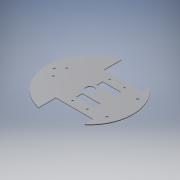
# Autodesk Inventor part: Base Inferior
Saved by Autodesk Inventor 2017 (Build 210142000, 142)
## iProperties
Created: 2017-08-05
Part Number: Base Inferior
Material: Glass
Document SubType Name: Modeling
Designer: Andre Rodas
Density: 2.18 g/cm^3
Appearance: Clear
Author: Andre Rodas
Autodesk Inventor part; units mm, degrees
ref_plane "YZ Plane" through (0, 0, 0) normal (1, 0, 0) x (0, 1, 0)
ref_plane "XZ Plane" through (0, 0, 0) normal (0, 1, 0) x (-1, 0, 0)
ref_plane "XY Plane" through (0, 0, 0) normal (0, 0, 1) x (1, 0, 0)
sketch "Sketch1" plane through (0, 0, 0) normal (0, 0, 1) x (1, 0, 0)
  circle A0 centre (0, 0) radius 50
  dimension "d0" = 100
  constraints: 1 centre point, 1 coincident
  measures "d0" diameter of A0
extrude "Extrusion1" add sketch "Sketch1" along normal blind 1
sketch "Sketch3" plane through (0, 0, 1) normal (0, 0, 1) x (1, 0, 0)
  circle A0 centre (0, 0) radius 50 construction
  line L0 (50, 0) -> (-50, 0)
  line L1 (10, 28) -> (-12, 28)
  line L2 (10, 28) -> (32, 28)
  line L3 (32, 28) -> (32, 38.4187)
  line L4 (-12, 28) -> (-12, 48.5386)
  line L5 (0, 0) -> (0, 50) construction
  arc A1 (32, 38.4187) -> (-12, 48.5386) centre (0, 0) ccw
  line L6 (32, -38.4187) -> (32, -28)
  line L7 (32, -28) -> (10, -28)
  line L8 (10, -28) -> (-12, -28)
  line L9 (-12, -28) -> (-12, -48.5386)
  line L10 (0, 0) -> (0, -50) construction
  arc A2 (-12, -48.5386) -> (32, -38.4187) centre (0, 0) ccw
  arc A3 (32, 38.4187) -> (-12, 48.5386) centre (0, 0) ccw
  dimension "d18" = 100
  dimension "d19" = 44
  dimension "d21" = 22
  dimension "d22" = 10
  dimension "d23" = 44
  dimension "d24" = 22
  dimension "d25" = 10
  constraints: 22 end point, 6 point on circle, 5 coincident, 3 centre point, 3 horizontal, 3 perpendicular, 3 vertical, 2 collinear, 1 midpoint, 1 parallel, 1 point on line, 11 other
  measures "d19" distance between parallel lines of L4 L3
  measures "d21" vertical distance of L5.end L1.start
  measures "d22" horizontal distance of L5.end L1.start
  measures "d23" distance between parallel lines of L9 L6
  measures "d24" vertical distance of L10.end L7.end
  measures "d25" horizontal distance of L10.end L7.end
extrude "Extrusion4" cut sketch "Sketch3" against normal through all
sketch "Sketch4" plane through (0, 0, 1) normal (0, 0, 1) x (1, 0, 0)
  line L0 (0, 0) -> (10, 0)
  line L1 (10, 0) -> (10, 12)
  line L2 (10, 0) -> (10, -12)
  line L3 (-0.75, -15.75) -> (20.75, -15.75)
  line L4 (20.75, -15.75) -> (20.75, -8.25)
  line L5 (20.75, -8.25) -> (-0.75, -8.25)
  line L6 (-0.75, -8.25) -> (-0.75, -15.75)
  line L7 (-0.75, -15.75) -> (20.75, -8.25) construction
  line L8 (20.75, -15.75) -> (-0.75, -8.25) construction
  line L9 (-0.75, 8.25) -> (20.75, 8.25)
  line L10 (20.75, 8.25) -> (20.75, 15.75)
  line L11 (20.75, 15.75) -> (-0.75, 15.75)
  line L12 (-0.75, 15.75) -> (-0.75, 8.25)
  line L13 (-0.75, 8.25) -> (20.75, 15.75) construction
  line L14 (20.75, 8.25) -> (-0.75, 15.75) construction
  dimension "d28" = 10
  dimension "d29" = 12
  dimension "d30" = 12
  dimension "d31" = 21.5
  dimension "d32" = 7.5
  dimension "d33" = 21.5
  dimension "d34" = 7.5
  constraints: 30 end point, 4 midpoint, 4 parallel, 3 horizontal, 2 perpendicular, 2 vertical
  measures "d28" distance of L0.start L0.end
  measures "d29" distance of L0.end L1.end
  measures "d30" distance of L0.end L2.end
  measures "d31" distance of L5.end L4.end
  measures "d32" distance of L4.end L3.end
  measures "d33" distance between parallel lines of L10 L12
  measures "d34" distance between parallel lines of L11 L9
extrude "Extrusion5" cut sketch "Sketch4" against normal through all
sketch "Sketch5" plane through (0, 0, 1) normal (0, 0, 1) x (1, 0, 0)
  circle A0 centre (0, 0) radius 5
  dimension "d37" = 10
  constraints: 1 centre point, 1 coincident
  measures "d37" diameter of A0
extrude "Extrusion6" cut sketch "Sketch5" against normal through all
sketch "Sketch6" plane through (0, 0, 1) normal (0, 0, 1) x (1, 0, 0)
  line L0 (20.75, -15.75) -> (-0.75, -15.75) projected
  line L1 (-0.75, 15.75) -> (20.75, 15.75) projected
  line L2 (20.75, 15.75) -> (-0.75, 15.75) projected
  line L3 (10, 15.75) -> (10, 21.75)
  line L4 (10, -15.75) -> (10, -21.75)
  line L5 (1.43, 21.75) -> (18.57, 21.75)
  line L6 (1.43, -21.75) -> (18.57, -21.75)
  circle A0 centre (1.43, 21.75) radius 1.25
  circle A1 centre (18.57, 21.75) radius 1.25
  circle A2 centre (1.43, -21.75) radius 1.25
  circle A3 centre (18.57, -21.75) radius 1.25
  point P0 (0, 0)
  dimension "d40" = 6
  dimension "d41" = 6
  dimension "d42" = 17.14
  dimension "d43" = 17.14
  dimension "d44" = 2.5
  dimension "d45" = 2.5
  dimension "d46" = 2.5
  dimension "d47" = 2.5
  constraints: 8 end point, 4 centre point, 4 coincident, 4 midpoint, 2 horizontal, 2 vertical
  measures "d40" distance of L3.end L3.start
  measures "d41" distance of L4.end L4.start
  measures "d42" distance of L5.start L5.end
  measures "d43" distance of L6.start L6.end
  measures "d44" diameter of A0
  measures "d45" diameter of A1
  measures "d46" diameter of A2
  measures "d47" diameter of A3
extrude "Extrusion7" cut sketch "Sketch6" against normal through all
sketch "Sketch7" plane through (0, 0, 1) normal (0, 0, 1) x (1, 0, 0)
  line L0 (0, 0) -> (-35, 0)
  line L1 (-35, -7.9) -> (-35, 7.9)
  circle A0 centre (-35, -7.9) radius 1.25
  circle A1 centre (-35, 7.9) radius 1.25
  dimension "d50" = 35
  dimension "d51" = 15.8
  dimension "d52" = 2.5
  dimension "d53" = 2.5
  constraints: 4 end point, 2 centre point, 2 coincident, 1 horizontal, 1 midpoint, 1 vertical
  measures "d50" distance of L0.end L0.start
  measures "d51" distance of L1.start L1.end
  measures "d52" diameter of A0
  measures "d53" diameter of A1
extrude "Extrusion8" cut sketch "Sketch7" against normal through all
sketch "Sketch8" plane through (0, 0, 1) normal (0, 0, 1) x (1, 0, 0)
  line L0 (0, 0) -> (-42, 0) construction
  line L1 (0, 0) -> (38, 0) construction
  line L2 (38, 0) -> (38, 18) construction
  line L3 (38, 0) -> (38, -18) construction
  circle A0 centre (-42, 0) radius 1.5
  circle A1 centre (38, 18) radius 1.5
  circle A2 centre (38, -18) radius 1.5
  dimension "d56" = 42
  dimension "d57" = 38
  dimension "d58" = 18
  dimension "d59" = 3
  constraints: 8 end point, 3 centre point, 3 coincident, 2 equal radius, 2 horizontal, 2 vertical, 1 collinear
  measures "d56" distance of L0.start L0.end
  measures "d57" distance of L0.start L1.end
  measures "d58" distance of L1.end L2.end
  measures "d59" diameter of A0
extrude "Extrusion9" cut sketch "Sketch8" against normal through all
equation "\"d23\" = d19"
equation "\"d24\" = d21"
equation "\"d25\" = d22"
equation "\"d28\" = d22"
equation "\"d29\" = d30"
equation "\"d33\" = d31"
equation "\"d34\" = d32"
equation "\"d38\" = d37"
equation "\"d43\" = d42"
body "Solid1"
